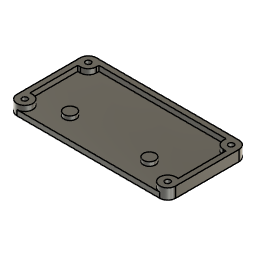
TRGRIP01_Base_Bottom_60x30x4 (Autodesk Fusion 360 design; units mm, degrees)
Autodesk Fusion 360 part; units mm, degrees
sketch "스케치1" plane through (0, 0, 0) normal (0, 0, 1) x (1, 0, 0)
  line L0 (0, 0) -> (60, 0)
  line L1 (60, 0) -> (60, 30)
  line L2 (60, 30) -> (0, 30)
  line L3 (0, 30) -> (0, 0)
  dimension "d1" = 60
  dimension "d2" = 30
  constraint horizontal L0
  constraint vertical L1
  constraint horizontal L2
  constraint vertical L3
  constraint coincident L0.start L3.end
  measures "d1" distance of L0.start L0.end
  measures "d2" distance of L0.start L2.end
extrude "돌출1" add sketch "스케치1" along normal blind 2
sketch "스케치5" plane through (0, 0, 2) normal (0, 0, 1) x (-1, 0, 0)
  line L0 (0, -30) -> (0, 0)
  line L1 (0, 0) -> (0, -30)
  line L2 (-60, -30) -> (0, -30)
  line L3 (-60, -30) -> (-60, 0)
  line L4 (0, 0) -> (-60, 0)
  line L5 (-60, 0) -> (-54, 0)
  line L6 (-54, -28) -> (-6, -28)
  line L7 (-2, -24) -> (-2, -6)
  line L8 (-6, 0) -> (0, 0)
  line L9 (-58, -24) -> (-58, -6)
  line L10 (-2, -24) -> (-6, -24)
  line L11 (-6, -24) -> (-6, -28)
  line L12 (-54, -28) -> (-54, -24)
  line L13 (-54, -24) -> (-58, -24)
  line L14 (-2, -6) -> (-6, -6)
  line L15 (0, 0) -> (-60, 0)
  line L16 (-6, -6) -> (-6, 0)
  line L17 (-58, -6) -> (-54, -6)
  line L18 (-54, -6) -> (-54, 0)
  point P0 (0, -30)
  point P1 (-60, -30)
  point P2 (-60, 0)
  dimension "d38" = 2
  dimension "d39" = 2
  dimension "d42" = 2
  dimension "d43" = 6
  dimension "d44" = 6
  dimension "d45" = 6
  dimension "d46" = 6
  dimension "d47" = 6
  constraint coincident L0.end L1.start
  constraint coincident P0 L0.start
  constraint coincident P1 L2.start
  constraint coincident P2 L3.end
  constraint coincident L4 L5.end
  constraint perpendicular L0 L5
  constraint perpendicular L0 L6
  constraint perpendicular L6 L7
  constraint perpendicular L1 L8
  constraint perpendicular L5 L9
  constraint perpendicular L7 L10
  constraint perpendicular L10 L11
  constraint perpendicular L6 L12
  constraint perpendicular L9 L13
  constraint perpendicular L7 L14
  constraint coincident L15 L8.start
  constraint perpendicular L15 L16
  constraint perpendicular L9 L17
  constraint perpendicular L4 L18
  constraint equal L10 L14
  constraint equal L11 L12
  constraint equal L13 L17
  measures "d38" distance of L2 L6
  measures "d39" distance of L3 L9
  measures "d42" distance of L1 L7
  measures "d43" distance of L0.end L8.start
  measures "d44" vertical distance of L0.end L14.end
  measures "d45" distance of P2 L5.end
  measures "d46" distance of L17.end L5.end
  measures "d47" vertical distance of P0 L10.end
extrude "돌출11" add sketch "스케치5" along normal blind 2 contours L0 L1 L2 L3 L4 L5 L6 L7 L8 L9 L10 L11 L12 L13 L14 L15 L16 L17 L18
sketch "스케치10" plane through (0, 0, 4) normal (0, 0, 1) x (-1, 0, 0)
  circle A0 centre (-57, -3) radius 1
  circle A1 centre (-57, -27) radius 1
  circle A2 centre (-3, -3) radius 1
  circle A3 centre (-3, -27) radius 1
  dimension "d82" = 2
  dimension "d83" = 3
  dimension "d84" = 3
  dimension "d85" = 24
  dimension "d86" = 54
  constraint equal A2 A3
  constraint equal A1 A2
  constraint equal A0 A1
  constraint vertical A2.centre A3.centre
  constraint horizontal A0.centre A2.centre
  constraint vertical A0.centre A1.centre
  constraint horizontal A1.centre A3.centre
  measures "d82" diameter of A0
  measures "d83" horizontal distance of origin A2.centre
  measures "d84" vertical distance of origin A2.centre
  measures "d85" distance of A2.centre A3.centre
  measures "d86" distance of A0.centre A2.centre
extrude "돌출13" cut sketch "스케치10" against normal blind 4
fillet "필렛4" radius 3 10 edges at (0, 0, 2) (60, 0, 2) (0, 30, 2) (60, 30, 2) (54, 24, 3) (6, 24, 3) (6, 6, 3) (54, 6, 3) (6, 0, 3) (54, 0, 3)
chamfer "챔퍼1" distance 1.5 angle 45 4 edges at (57.9323, 3.3616, 0) (57.9323, 27.3616, 0) (3.9323, 27.3616, 0) (3.9323, 3.3616, 0)
sketch "스케치11" plane through (0, 0, 2) normal (0, 0, 1) x (-1, 0, 0)
  circle A0 centre (-45, -8.1) radius 2.3
  circle A1 centre (-15, -8.1) radius 2.3
  dimension "d93" = 8.1
  dimension "d95" = 4.6
  dimension "d98" = 15
  dimension "d99" = 30
  constraint equal A0 A1
  constraint horizontal A0.centre A1.centre
  measures "d93" vertical distance of origin A0.centre
  measures "d95" diameter of A0
  measures "d98" horizontal distance of origin A1.centre
  measures "d99" distance of A0.centre A1.centre
extrude "돌출14" add sketch "스케치11" along normal blind 1.5
